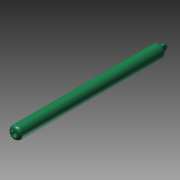
# Autodesk Inventor part: piston_outer
Saved by Autodesk Inventor 2012 (Build 160160000, 160)
## iProperties
Created: 2011-12-02
Part Number: piston_outer
Material: Default
Document SubType Name: Modeling
Designer: Antonella
Density: 1 g/cm^3
Author: Antonella
Autodesk Inventor part; units mm, degrees
ref_plane "YZ Plane" through (0, 0, 0) normal (1, 0, 0) x (0, 1, 0)
ref_plane "XZ Plane" through (0, 0, 0) normal (0, 1, 0) x (-1, 0, 0)
ref_plane "XY Plane" through (0, 0, 0) normal (0, 0, 1) x (1, 0, 0)
sketch "Sketch1" plane through (0, 0, 0) normal (0, 0, 1) x (1, 0, 0)
  circle A0 centre (0, 0) radius 6.35
  dimension "d0" = 12.7
  constraints: 1 centre point, 1 coincident
  measures "d0" diameter of A0
extrude "Extrusion1" add sketch "Sketch1" along normal mid plane 152.4
sketch "Sketch2" plane through (0, 0, 76.2) normal (0, 0, 1) x (1, 0, 0)
  circle A0 centre (0, 0) radius 6.35 projected
  circle A1 centre (0, 0) radius 3.175
  dimension "d3" = 6.35
  constraints: 1 centre point, 1 coincident
  measures "d3" diameter of A1
extrude "Extrusion2" cut sketch "Sketch2" against normal blind 139.7 contours A1
fillet "Fillet1" radius 3.175 2 edges at (-6.35, 0, -76.2) (-6.35, 0, 76.2)
sketch "Sketch3" plane through (0, 0, -76.2) normal (0, 0, -1) x (-1, 0, 0)
  circle A0 centre (0, 0) radius 3.175 projected
  line L0 (-1.1906, 2.9433) -> (-1.1906, -2.9433)
  line L1 (1.1906, 2.9433) -> (1.1906, -2.9433)
  line L2 (0, -8.89) -> (0, 8.89) projected
  line L3 (-1.1906, 2.9433) -> (1.1906, 2.9433)
  line L4 (1.1906, -2.9433) -> (-1.1906, -2.9433)
  dimension "d7" = 2.3813
  constraints: 8 end point, 4 point on circle, 2 parallel, 1 perpendicular, 1 vertical
  measures "d7" distance between parallel lines of L0 L1
extrude "Extrusion3" add sketch "Sketch3" along normal blind 6.35 contours L1 L4 L2 L3 | L2 L4 L0 L3
sketch "Sketch4" plane through (-1.1906, -2.9433, -76.2) normal (-1, 0, 0) x (0, 0, 1)
  line L0 (-6.35, 5.8866) -> (-6.35, 0) projected
  line L1 (0, 0) -> (-6.35, 0) projected
  line L2 (0, 5.8866) -> (0, 0) projected
  line L3 (0, 5.8866) -> (-6.35, 5.8866) projected
  arc A0 (-3.4067, 5.8866) -> (-3.4067, 0) centre (-3.4067, 2.9433) ccw
  point P0 (76.2, 2.9433)
  constraints: 3 tangent, 2 point on circle, 2 point on line, 1 centre point
extrude "Extrusion4" cut sketch "Sketch4" against normal through all contours L3 A0 L0 | A0 L1 L0
body "Solid1"
